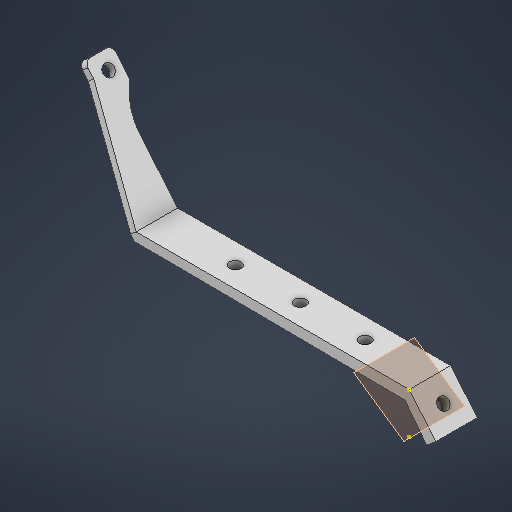
# Autodesk Inventor part: для жгутов2 ipt
Saved by Autodesk Inventor 2026.2 (Build 302298000, 298)
## iProperties
Created: 2026-01-08
Part Number: для жгутов2 ipt
Material: Типовые
Document SubType Name: Modeling
Designer: Phantom_HP2
Density: 1 g/cm^3
Appearance: По умолчанию
Author: Phantom_HP2
Autodesk Inventor part; units mm, degrees
ref_plane "YZ Plane" through (0, 0, 0) normal (1, 0, 0) x (0, 1, 0)
ref_plane "XZ Plane" through (0, 0, 0) normal (0, 1, 0) x (-1, 0, 0)
ref_plane "XY Plane" through (0, 0, 0) normal (0, 0, 1) x (1, 0, 0)
sketch "Эскиз1" plane through (0, 0, 0) normal (0, 1, 0) x (-1, 0, 0)
  line L0 (0, 0) -> (140.8, 0)
  line L1 (140.8, 0) -> (140.8, -15)
  line L2 (140.8, -15) -> (0, -15)
  circle A0 centre (23.47, -7.5) radius 2.1
  circle A1 centre (46.94, -7.5) radius 2.1
  circle A2 centre (70.41, -7.5) radius 2.1
  circle A3 centre (93.86, -7.5) radius 2.1
  circle A4 centre (117.33, -7.5) radius 2.1
  line L3 (0, 0) -> (0, -15)
  dimension "d1" = 15
  dimension "d2" = 140.8
  dimension "d3" = 4.2
  dimension "d5" = 7.5
  dimension "d6" = 4.2
  dimension "d8" = 4.2
  dimension "d10" = 4.2
  dimension "d12" = 4.2
  dimension "d14" = 23.47
  dimension "d16" = 23.47
  dimension "d17" = 23.47
  dimension "d18" = 23.47
  constraints: 8 end point, 5 centre point, 1 horizontal, 1 parallel, 1 perpendicular, 1 vertical
  measures "d1" distance of L0.end L1.end
  measures "d2" distance of L1.end L2.end
  measures "d3" diameter of A0
  measures "d5" distance from line of L2 A0.centre
  measures "d6" diameter of A1
  measures "d8" diameter of A2
  measures "d10" diameter of A3
  measures "d12" diameter of A4
  measures "d14" distance from line of L1 A4.centre
  measures "d16" distance of A1.centre A0.centre
  measures "d17" distance of A4.centre A3.centre
  measures "d18" distance of A1.centre A2.centre
extrude "Выдавливание1" add sketch "Эскиз1" along normal blind 15
sketch "Эскиз7" plane through (-140.8, 0, -15) normal (0, 0, -1) x (-1, 0, 0)
  line L0 (-155.8, -0.8981) -> (-138.4224, 11.7275) projected
  line L1 (-140.8, 15) -> (-93.6153, -51.5286)
  line L2 (-93.6153, -51.5286) -> (0.1874, 15)
  line L3 (-140.8, 15) -> (0, 15) projected
  line L4 (-20.962, 0) -> (0, 0)
  line L5 (0, 0) -> (0, 15)
  line L6 (-140.8, 15) -> (0, 15)
  line L7 (-20.962, 0) -> (0, 0)
  line L8 (0.1874, 15) -> (0.1874, 0)
  line L9 (0, 0) -> (0, 15) projected
  point P0 (-140.8, 0)
  point P1 (0, 14.8671)
  dimension "d50" = 81.5625
  dimension "d51" = 115
  dimension "d52" = 0
  constraints: 14 end point, 3 perpendicular, 2 point on line, 1 collinear, 1 horizontal, 1 vertical, 1 other
  measures "d50" distance of L0.end L1.end
  measures "d51" distance of L1.end L2.end
  measures "d52" distance from line of L3 L2.end
extrude "Выдавливание6" cut sketch "Эскиз7" against normal blind 15 contours L5 L4 L2
sketch "Эскиз8" plane through (0, 15, -15) normal (0, 0, -1) x (-1, 0, 0)
  line L0 (0, 0) -> (140.8, 0) projected
  line L1 (0, 0) -> (36.7423, -59.5819)
  line L2 (36.7423, -59.5819) -> (123.5616, -6.0432)
  line L3 (0, 0) -> (-29.0636, -18.4877)
  circle A0 centre (123.5616, -6.0432) radius 2.1
  point P0 (0, -15)
  dimension "d55" = 70
  dimension "d56" = 102
  dimension "d76" = 4.2
  constraints: 6 end point, 1 centre point, 1 coincident, 1 perpendicular
  measures "d55" distance of L0.start L1.end
  measures "d56" distance of L1.end L2.end
  measures "d76" diameter of A0
ref_plane "РабПлоскость1" through (0, 15, 0) normal (0.5658425, 0.8245133, 0) x (0.8245133, -0.5658425, 0)
sketch "Эскиз10" plane through (0, 15, 0) normal (0.5658425, 0.8245133, 0) x (0.8245133, -0.5658425, 0)
  circle A0 centre (18.4448, 7.5) radius 2.1
  line L0 (25.9448, 0) -> (0, 0) projected
  line L1 (25.9448, 15) -> (25.9448, 0) projected
  point P0 (8.4876, 0)
  dimension "d69" = 4.2
  dimension "d70" = 7.5
  dimension "d71" = 7.5
  constraints: 1 centre point
  measures "d69" diameter of A0
  measures "d70" distance from line of L0 A0.centre
  measures "d71" distance from line of L1 A0.centre
extrude "Выдавливание9" cut sketch "Эскиз10" against normal blind 15
sketch "Эскиз11" plane through (0, 15, 0) normal (0, 1, 0) x (1, 0, 0)
  point P0 (0, 0)
sketch "Эскиз12" plane through (0, 15, 0) normal (0, 1, 0) x (1, 0, 0)
  circle A0 centre (-23.47, 7.5) radius 2.1 projected
  circle A1 centre (-46.94, 7.5) radius 2.1 projected
  circle A2 centre (-70.41, 7.5) radius 2.1 projected
  circle A3 centre (-93.86, 7.5) radius 2.1 projected
  circle A4 centre (-117.33, 7.5) radius 2.1 projected
  point P0 (0, 0)
extrude "Выдавливание10" cut sketch "Эскиз12" against normal blind 15
extrude "Выдавливание11" cut sketch "Эскиз8" against normal blind 15
sketch "Эскиз13" plane through (-140.8, 15, 0) normal (0, 0, 1) x (1, 0, 0)
  point P0 (140.8, -15)
sketch "Эскиз14" plane through (-140.8, 15, 0) normal (0, 0, 1) x (1, 0, 0)
  line L0 (140.8, 0) -> (0, 0) projected
  line L1 (0, 0) -> (-37, 0)
  line L2 (-37, 0) -> (-15.8506, -15)
  line L3 (-15.8506, -15) -> (6.9783, -15)
  line L4 (0, -0.1329) -> (20.962, -15) projected
  line L5 (0, -0.1329) -> (20.962, -15)
  line L6 (6.9783, -15) -> (20.962, -15)
  point P0 (140.8, -15)
  dimension "d79" = 37
  constraints: 10 end point, 2 horizontal, 2 parallel, 1 collinear, 1 point on line
  measures "d79" distance of L0.end L1.end
extrude "Выдавливание12" add sketch "Эскиз14" against normal blind 15 fills toward (70.4, -0.05) open curves L0 L1 L2 L3 L6
sketch "Эскиз15" plane through (-177.8, 15, 0) normal (0, 0, 1) x (1, 0, 0)
  line L0 (199.1918, -14.6807) -> (189.9964, -28.0798) projected
  line L1 (196.7887, -18.1824) -> (176.257, -4.092)
  line L2 (176.257, -4.092) -> (-2.2045, -2.6356)
  line L3 (-2.2045, -2.6356) -> (22.7303, -26.1279)
  line L4 (22.7303, -26.1279) -> (189.9964, -36.2255)
  line L5 (189.9964, -36.2255) -> (196.7887, -18.1824)
  point P0 (177.8, -15)
  constraints: 10 end point, 1 perpendicular, 1 point on line
extrude "Выдавливание13" cut sketch "Эскиз15" against normal blind 8
sketch "Эскиз16" plane through (-177.8, 15, -8) normal (0, 0, 1) x (1, 0, 0)
  point P0 (177.8, -15)
sketch "Эскиз17" plane through (-177.8, 15, -8) normal (0, 0, 1) x (1, 0, 0)
  line L0 (3.7851, -2.6845) -> (176.257, -4.092) projected
  line L1 (176.257, -4.092) -> (177.8, -5.1509) projected
  line L2 (3.7851, -2.6845) -> (176.257, -4.092)
  line L3 (176.257, -4.092) -> (214.4439, -30.2987)
  line L4 (214.4439, -30.2987) -> (97.3846, -64.0666)
  line L5 (97.3846, -64.0666) -> (-1.4773, -35.1954)
  line L6 (-1.4773, -35.1954) -> (3.7851, -2.6845)
  point P0 (177.8, -15)
  point P1 (188.9232, -12.7845)
  constraints: 10 end point, 1 collinear
extrude "Выдавливание14" cut sketch "Эскиз17" against normal blind 8
sketch "Эскиз18" plane through (-177.8, 15, 0) normal (0, 0, 1) x (1, 0, 0)
  line L0 (177.8, 0) -> (199.1918, -14.6807) projected
  line L1 (177.8, 0) -> (176.257, -4.092)
  line L2 (176.257, -4.092) -> (193.5103, -30.0978)
  line L3 (193.5103, -30.0978) -> (209.0736, -14.129)
  line L4 (209.0736, -14.129) -> (177.8, 0)
  point P0 (177.8, -15)
  constraints: 8 end point
extrude "Выдавливание15" cut sketch "Эскиз18" against normal blind 15
sketch "Эскиз21" plane through (-177.8, 15, 0) normal (0, 0, 1) x (1, 0, 0)
  line L0 (177.8, 0) -> (0, 0) projected
  line L1 (177.8, 0) -> (189.9353, -8.8168)
  line L2 (177.8, 0) -> (176.257, -4.092) projected
  line L3 (176.257, -4.092) -> (187.4563, -12.2288)
  line L4 (189.9353, -8.8168) -> (187.4563, -12.2288)
  point P0 (177.8, -15)
  dimension "d92" = 15
  dimension "d94" = 36
  constraints: 6 end point, 1 parallel, 1 perpendicular
  measures "d92" distance of L0.start L1.end
  measures "d94" angle of L0 L1
extrude "Выдавливание17" add sketch "Эскиз21" against normal blind 15
sketch "Эскиз22" plane through (12.1353, 6.1832, 0) normal (0.5877853, 0.809017, 0) x (0.809017, -0.5877853, 0)
  circle A0 centre (-7.5, 7.5) radius 2.1
  line L0 (-15, 15) -> (0, 15) projected
  line L1 (0, 0) -> (0, 15) projected
  point P0 (-6.1832, 0)
  dimension "d97" = 4.2
  dimension "d98" = 7.5
  dimension "d99" = 7.5
  constraints: 1 centre point
  measures "d97" diameter of A0
  measures "d98" distance from line of L0 A0.centre
  measures "d99" distance from line of L1 A0.centre
extrude "Выдавливание18" cut sketch "Эскиз22" against normal blind 15
sketch "Эскиз23" plane through (-177.8, 15, 0) normal (0, 0, 1) x (1, 0, 0)
  line L0 (189.9353, -8.8168) -> (177.8, 0) projected
  line L1 (186.549, -103.0788) -> (-44.6132, 64.8703)
  line L2 (-44.6132, 64.8703) -> (-26.2742, -77.5538)
  line L3 (-26.2742, -77.5538) -> (186.549, -103.0788)
  point P0 (177.8, -15)
  dimension "d106" = 78.25
  constraints: 6 end point, 1 parallel
  measures "d106" distance between parallel lines of L0 L1
extrude "Выдавливание19" cut sketch "Эскиз23" against normal blind 15
sketch "Эскиз24" plane through (-133.1269, 15, 0) normal (0, 0, 1) x (1, 0, 0)
  line L0 (133.1269, 0) -> (0, 0) projected
  line L1 (12.3018, 0) -> (7.7798, -5.6524)
  line L2 (4.2014, -3.0525) -> (131.5839, -4.092) projected
  line L3 (0, 0) -> (4.2014, -3.0525) projected
  line L4 (0, 0) -> (7.7798, -5.6524)
  line L5 (12.3018, 0) -> (9.3018, 0)
  line L6 (0, 0) -> (3, 0)
  line L7 (145.2621, -8.8168) -> (133.1269, 0) projected
  line L8 (12.3018, 0) -> (0, 0)
  point P0 (133.1269, -15)
  constraints: 10 end point, 3 point on line, 2 collinear, 1 parallel
extrude "Выдавливание20" cut sketch "Эскиз24" against normal blind 15
sketch "Эскиз25" plane through (-120.8251, 15, 0) normal (0, 0, 1) x (1, 0, 0)
  line L0 (120.8251, 0) -> (0, 0) projected
  line L1 (0, 0) -> (-7.231, -9.9526)
  line L2 (-7.231, -9.9526) -> (-17.231, -2.6872)
  line L3 (132.9603, -8.8168) -> (120.8251, 0) projected
  line L4 (-17.231, -2.6872) -> (-14.8799, 0.5489)
  line L5 (-14.8799, 0.5489) -> (-8.8799, -3.8363)
  line L6 (-8.8799, -3.8363) -> (-6.0761, 0)
  line L7 (-6.0761, 0) -> (0, 0)
  point P0 (120.8251, -15)
  dimension "d113" = 7.231
  dimension "d114" = 10
  dimension "d115" = 4
  dimension "d117" = 6
  constraints: 12 end point, 2 parallel, 2 perpendicular, 1 horizontal
  measures "d113" horizontal distance of L0.end L1.end
  measures "d114" horizontal distance of L1.end L2.end
  measures "d115" distance of L2.end L4.end
  measures "d117" horizontal distance of L4.end L5.end
extrude "Выдавливание21" add sketch "Эскиз25" against normal blind 15
sketch "Эскиз26" plane through (-126.9012, 15, 0) normal (0, 0, 1) x (1, 0, 0)
  line L0 (136.5575, -12.2288) -> (125.3582, -4.092) projected
  line L1 (126.9012, 0) -> (125.3582, -4.092)
  line L2 (125.3582, -4.092) -> (134.8995, -15)
  line L3 (134.8995, -15) -> (146, -9)
  line L4 (146, -9) -> (126.9012, 0)
  point P0 (126.9012, -15)
  constraints: 8 end point
extrude "Выдавливание22" cut sketch "Эскиз26" against normal blind 15
sketch "Эскиз27" plane through (-126.9012, 15, 0) normal (0, 0, 1) x (1, 0, 0)
  line L0 (0, 0) -> (126.9012, 0) projected
  line L1 (126.9012, 0) -> (136.543, -11.4907)
  line L2 (125.3582, -4.092) -> (3.8237, -3.1002) projected
  line L3 (125.3582, -4.092) -> (133, -14)
  line L4 (136.543, -11.4907) -> (133.2171, -14.2814)
  line L5 (133, -14) -> (133.2171, -14.2814)
  line L6 (125.3582, -4.092) -> (126.9012, 0)
  point P0 (126.9012, -15)
  dimension "d122" = 15
  dimension "d123" = 50
  constraints: 10 end point, 1 collinear, 1 perpendicular
  measures "d122" distance of L0.end L1.end
  measures "d123" angle of L0 L1
extrude "Выдавливание23" add sketch "Эскиз27" against normal blind 15
sketch "Эскиз28" plane through (0, 15, 0) normal (0, 1, 0) x (1, 0, 0)
  circle A0 centre (-117.33, 7.5) radius 2.1
  circle A1 centre (-117.33, 7.5) radius 2.1 projected
  point P0 (0, 0)
  dimension "d126" = 4.2
  constraints: 1 centre point, 1 concentric
  measures "d126" diameter of A0
extrude "Выдавливание24" add sketch "Эскиз28" against normal up to surface surface through (-180.0045, 12.3644, 0) normal (0.0081606, 0.9999667, 0)
sketch "Эскиз29" plane through (-126.9012, 15, 0) normal (0, 0, 1) x (1, 0, 0)
  line L0 (8, 12) -> (33.7662, -21.4071)
  line L1 (125.3582, -4.092) -> (133.2171, -14.2814) projected
  line L2 (8, 12) -> (-38, 2)
  line L3 (-38, 2) -> (-2.8789, -29.3734)
  line L4 (-2.8789, -29.3734) -> (33.7662, -21.4071)
  point P0 (126.9012, -15)
  constraints: 8 end point, 2 parallel
extrude "Выдавливание25" cut sketch "Эскиз29" against normal blind 15
sketch "Эскиз30" plane through (-109.6458, 15, 0) normal (0, 0, 1) x (1, 0, 0)
  point P0 (109.6458, -15)
sketch "Эскиз31" plane through (0, 15, 0) normal (0, 1, 0) x (1, 0, 0)
  point P0 (0, 0)
sketch "Эскиз32" plane through (-109.6458, 15, 0) normal (0, 0, 1) x (1, 0, 0)
  line L0 (13.6858, 0) -> (17.8858, 0) projected
  line L1 (17.8858, 0) -> (14, 14)
  line L2 (14, 14) -> (-6, 8)
  line L3 (-6, 8) -> (-3, -12)
  line L4 (-3, -12) -> (32.7763, -11.836)
  line L5 (17.8858, 0) -> (26.2705, -11.8658)
  point P0 (109.6458, -15)
  constraints: 10 end point, 1 equal length, 1 point on line
extrude "Выдавливание26" cut sketch "Эскиз32" against normal blind 15
sketch "Эскиз33" plane through (-91.76, 15, 0) normal (0, 0, 1) x (1, 0, 0)
  line L0 (0, 0) -> (91.76, 0) projected
  line L1 (0, 0) -> (-10, 0)
  line L2 (0, 0) -> (2.385, -3.3753) projected
  line L3 (2.385, -3.3753) -> (-7.615, -3.3753)
  line L4 (-10, 0) -> (-7.615, -3.3753)
  point P0 (91.76, -15)
  dimension "d133" = 10
  constraints: 6 end point, 2 horizontal, 1 parallel
  measures "d133" distance of L0.start L1.end
extrude "Выдавливание27" add sketch "Эскиз33" against normal up to surface (15 mm away)
sketch "Эскиз34" plane through (-101.76, 15, 0) normal (0, 0, 1) x (1, 0, 0)
  line L0 (0, 0) -> (101.76, 0) projected
  line L1 (0, 0) -> (-21.6938, 30.7008)
  line L2 (0, 0) -> (2.385, -3.3753) projected
  line L3 (-21.6938, 30.7008) -> (-19.6938, 32.114)
  line L4 (-19.6938, 32.114) -> (2.9986, 0)
  line L5 (0, 0) -> (2.9986, 0)
  point P0 (101.76, -15)
  dimension "d136" = 37.592
  dimension "d137" = 2
  constraints: 8 end point, 2 collinear, 2 perpendicular, 1 point on line
  measures "d136" distance of L0.start L1.end
  measures "d137" horizontal distance of L1.end L3.end
extrude "Выдавливание28" add sketch "Эскиз34" against normal up to surface (15 mm away)
sketch "Эскиз35" plane through (-99.375, 11.6247, 0) normal (0, 0, 1) x (1, 0, 0)
  point P0 (99.375, -11.6247)
sketch "Эскиз36" plane through (-99.375, 11.6247, 0) normal (0, 0, 1) x (1, 0, 0)
  line L0 (-24.0789, 34.076) -> (0, 0) projected
  line L1 (0, 0) -> (-26.9104, 32.0752)
  line L2 (-22.0789, 35.4892) -> (-24.0789, 34.076) projected
  line L3 (-24.0789, 34.076) -> (-26.9104, 32.0752)
  line L4 (-24.0789, 34.076) -> (0, 0)
  point P0 (99.375, -11.6247)
  dimension "d140" = 4.75
  constraints: 6 end point, 2 collinear, 1 point on line
  measures "d140" angle of L0 L1
extrude "Выдавливание29" add sketch "Эскиз36" against normal up to surface (15 mm away)
sketch "Эскиз37" plane through (-98.7614, 15, 0) normal (0, 0, 1) x (1, 0, 0)
  line L0 (0, 0) -> (-22.6925, 32.114) projected
  line L1 (-22.6925, 32.114) -> (0, 0)
  line L2 (0, 0) -> (-25.3609, 30.2284)
  line L3 (-22.6925, 32.114) -> (-27.524, 28.7) projected
  point P0 (98.7614, -15)
  dimension "d143" = 4.75
  constraints: 4 end point, 1 collinear, 1 point on line
  measures "d143" angle of L2 L0
extrude "Выдавливание30" cut sketch "Эскиз37" against normal up to surface (15 mm away)
sketch "Эскиз38" plane through (-124.1223, 45.2284, 0) normal (0.7660908, 0.6427324, 0) x (0, 0, -1)
  line L0 (20, 5.2193) -> (10, 5.2193)
  line L1 (10, 5.2193) -> (10, -4.7807)
  line L2 (10, -4.7807) -> (20, -4.7807)
  line L3 (20, -4.7807) -> (20, 5.2193)
  line L4 (0, 0.2193) -> (15, 0.2193) projected
  line L5 (20, 5.2193) -> (10, -4.7807) construction
  line L6 (10, 5.2193) -> (20, -4.7807) construction
  point P0 (0, -114.4265)
  dimension "d146" = 10
  dimension "d147" = 10
  constraints: 12 end point, 2 midpoint, 2 parallel, 1 horizontal, 1 perpendicular
  measures "d146" distance of L2.end L1.end
  measures "d147" distance of L1.end L0.end
extrude "Выдавливание31" add sketch "Эскиз38" against normal up to surface (2.6395 mm away)
sketch "Эскиз39" plane through (-98.7614, 15, 0) normal (0.7660908, 0.6427324, 0) x (0, 0, -1)
  line L0 (15, 0) -> (0, 0) projected
  line L1 (10, 39.458) -> (0, 0)
  line L2 (0, 0) -> (0, 39.458)
  line L3 (0, 39.458) -> (10, 39.458)
  line L4 (10, 39.458) -> (4.7946, 43.4178)
  line L5 (4.7946, 43.4178) -> (-2.7711, 41.5661)
  line L6 (-2.7711, 41.5661) -> (0, 39.458)
  point P0 (0, -74.9685)
  constraints: 12 end point, 2 perpendicular, 1 parallel
extrude "Выдавливание32" cut sketch "Эскиз39" against normal blind 10
fillet "Сопряжение1" radius 19.75 1 edges at (-122.0606, 40.7177, -15)
fillet "Сопряжение2" radius 2 3 edges at (-128.488, 48.3786, -10) (-128.488, 48.3786, -20) (-122.0606, 40.7177, -20)
sketch "Эскиз40" plane through (-98.7614, 15, 0) normal (0.7660908, 0.6427324, 0) x (0, 0, -1)
  line L0 (9.7117, 39.6773) -> (10, 39.458) projected
  line L1 (9.7117, 39.6773) -> (10, 39.458) projected
  line L2 (10, 39.458) -> (10, 39.6773) projected
  line L3 (9.7117, 39.6773) -> (10, 39.6773) projected
  point P0 (0, -74.9685)
extrude "Выдавливание33" cut sketch "Эскиз40" against normal blind 10
sketch "Эскиз41" plane through (9.6418, 3.5093, 0) normal (0.7660444, 0.6427876, 0) x (0, 0, -1)
  circle A0 centre (7.5, 7.5) radius 2.1
  line L0 (0, 0) -> (15, 0) projected
  line L1 (15, 15) -> (15, 0) projected
  point P0 (0, 3.5093)
  dimension "d156" = 4.2
  dimension "d157" = 7.5
  dimension "d158" = 7.5
  constraints: 1 centre point
  measures "d156" diameter of A0
  measures "d157" distance from line of L0 A0.centre
  measures "d158" distance from line of L1 A0.centre
extrude "Выдавливание34" cut sketch "Эскиз41" against normal blind 10
sketch "Эскиз42" plane through (-98.7614, 15, 0) normal (0.7660908, 0.6427324, 0) x (0, 0, -1)
  circle A0 centre (15.397, 39.5173) radius 2.1
  line L0 (18, 44.6773) -> (12, 44.6773) projected
  line L1 (20, 35.4178) -> (20, 42.6773) projected
  point P0 (0, -74.9685)
  dimension "d161" = 4.2
  dimension "d162" = 5.16
  dimension "d163" = 4.603
  constraints: 1 centre point
  measures "d161" diameter of A0
  measures "d162" distance from line of L0 A0.centre
  measures "d163" distance from line of L1 A0.centre
extrude "Выдавливание35" cut sketch "Эскиз42" against normal blind 10
